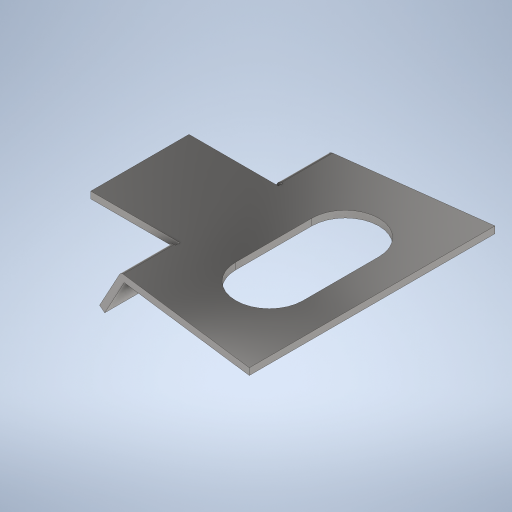
# Autodesk Inventor part: MK_5_rust_helma
Saved by Autodesk Inventor 2023 (Build 270158000, 158)
## iProperties
Created: 2025-04-03
Part Number: MK_5_rust_helma
Material: Všeobecné
Document SubType Name: Modeling
Designer: kolom_rupe2o
Density: 1 g/cm^3
Appearance: Ocel – leštěná
Author: kolom_rupe2o
Autodesk Inventor part; units mm, degrees
ref_plane "YZ Plane" through (0, 0, 0) normal (1, 0, 0) x (0, 1, 0)
ref_plane "XZ Plane" through (0, 0, 0) normal (0, 1, 0) x (-1, 0, 0)
ref_plane "XY Plane" through (0, 0, 0) normal (0, 0, 1) x (1, 0, 0)
sketch "Náčrt1" plane through (0, 0, 0) normal (0, 1, 0) x (-1, 0, 0)
  line L0 (0, 0) -> (0, -55)
  line L1 (0, -55) -> (32, -51)
  line L2 (32, -51) -> (32, -4)
  line L3 (32, -4) -> (0, 0)
  line L4 (14.5, -19) -> (14.5, -36) construction
  line L5 (7, -19) -> (7, -36)
  line L6 (22, -36) -> (22, -19)
  arc A0 (22, -19) -> (7, -19) centre (14.5, -19) ccw
  arc A1 (7, -36) -> (22, -36) centre (14.5, -36) ccw
  line L7 (32, -16.5) -> (52, -16.5)
  line L8 (52, -16.5) -> (52, -38.5)
  line L9 (52, -38.5) -> (32, -38.5)
  line L10 (32, -38.5) -> (32, -16.5)
  point P0 (32, -27.5)
  point P1 (0, -27.5)
  point P2 (14.5, -27.5)
  point P3 (52, -27.5)
  dimension "d0" = 47
  dimension "d1" = 55
  dimension "d2" = 32
  dimension "d3" = 10
  dimension "d4" = 7.5
  dimension "d5" = 17
  dimension "d6" = 22
  dimension "d7" = 20
  constraints: 24 end point, 4 midpoint, 4 parallel, 4 point on circle, 4 tangent, 3 horizontal alignment, 2 centre point, 2 vertical, 1 equal length, 1 horizontal, 1 perpendicular, 1 point on line
  measures "d0" distance of L1.end L2.end
  measures "d1" distance of L0.start L0.end
  measures "d2" distance between parallel lines of L0 L2
  measures "d3" distance between parallel lines of L2 L6
  measures "d4" radius of A1
  measures "d5" distance of L4.start L4.end
  measures "d6" distance of L7.end L8.end
  measures "d7" distance of L8.end L9.end
extrude "Vysunutí1" add sketch "Náčrt1" along normal blind 1.5
ref_plane "Pracovní rovina1" through (-52, 0, -27.5) normal (0, 0, 1) x (1, 0, 0)
ref_plane "Pracovní rovina2" through (-52, 0, -15.5) normal (0, 0, 1) x (1, 0, 0)
sketch "Náčrt3" plane through (-52, 0, -15.5) normal (0, 0, 1) x (1, 0, 0)
  line L0 (20, 0) -> (52, 0) projected
  line L1 (52, 0) -> (52, 1.5) projected
  line L2 (20, 1.5) -> (52, 1.5) projected
  line L3 (20, 0) -> (20, 1.5) projected
  line L4 (20, 0) -> (15, -8.6603)
  line L5 (15, -8.6603) -> (13.701, -7.9103)
  line L6 (13.701, -7.9103) -> (19.134, 1.5)
  line L7 (19.134, 1.5) -> (20, 1.5)
  line L8 (20, 0) -> (20, 1.5) projected
  line L9 (20, 0) -> (20, 1.5) projected
  dimension "d14" = 120
  dimension "d15" = 1.5
  dimension "d16" = 10
  constraints: 8 end point, 2 perpendicular, 1 collinear
  measures "d14" angle of L0 L4
  measures "d15" distance of L4.end L5.end
  measures "d16" distance of L0.start L4.end
extrude "Vysunutí2" add sketch "Náčrt3" along normal up to surface contours L4 L5 L6 L7 L3 surface through (-32, 0, -4) normal (-0.1240347, 0, 0.9922779)
sketch "Náčrt4" plane through (-32.866, 1.5, -15.5) normal (-0.8660254, 0.5, 0) x (0, 0, 1)
  line L0 (10.7126, -10.866) -> (11.3917, 0) projected
  line L1 (0, 0) -> (11.3917, 0) projected
  line L2 (0, 0) -> (0, -10.866) projected
  line L3 (0, -10.866) -> (10.7126, -10.866) projected
  point P0 (15.5, 15.134)
  point P1 (5.3563, -5.433)
  point P2 (0, -5.433)
  point P3 (5.3563, -10.866)
  constraints: 2 midpoint, 1 horizontal alignment, 1 vertical alignment
hole "Díra1" at (-35.5825, -3.2051, -10.1437) direction (0.8660254, -0.5, 0) diameter 3 end through all
mirror "Zrcadlit1" about plane through (-52, 0, -27.5) normal (0, 0, 1) of "Díra1", "Vysunutí2"
fillet "Zaoblení1" radius 1 2 edges at (-32.866, 1.5, -45.1959) (-32.866, 1.5, -9.8041)
